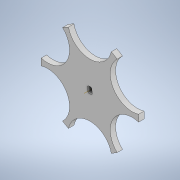
# Autodesk Inventor part: шестеренка_для_мозговорота
Saved by Autodesk Inventor 2021.1 (Build 251245010, 245A)
## iProperties
Created: 2022-11-11
Part Number: шестеренка_для_мозговорота
Material: Типовые
Document SubType Name: Modeling
Designer: zmoze
Density: 1 g/cm^3
Appearance: По умолчанию
Author: zmoze
Autodesk Inventor part; units mm, degrees
ref_plane "YZ Plane" through (0, 0, 0) normal (1, 0, 0) x (0, 1, 0)
ref_plane "XZ Plane" through (0, 0, 0) normal (0, 1, 0) x (-1, 0, 0)
sketch "Эскиз1" plane through (0, 0, 0) normal (0, 0, 1) x (1, 0, 0)
  arc A0 (-19.7308, 40.4437) -> (19.7308, 40.4437) centre (0, 0) ccw
  circle A1 centre (0, 45) radius 20.25
  line L0 (0, 91.35) -> (0, -91.35) projected
  circle A2 centre (-38.9711, 22.5) radius 20.25
  circle A3 centre (-38.9711, -22.5) radius 20.25
  circle A4 centre (0, -45) radius 20.25
  circle A5 centre (38.9711, -22.5) radius 20.25
  circle A6 centre (38.9711, 22.5) radius 20.25
  point P0 (-19.7308, -40.4437)
  point P1 (19.7308, -40.4438)
  point P2 (25.1599, -37.3092)
  point P3 (44.8907, -3.1345)
  point P4 (44.8907, 3.1345)
  point P5 (25.1599, 37.3092)
  point P6 (-25.1599, 37.3092)
  point P7 (-44.8907, 3.1345)
  point P8 (-44.8907, -3.1345)
  point P9 (-25.1599, -37.3092)
  dimension "d0" = 40.5
  dimension "d3" = 360
  dimension "d5" = 90
  constraints: 7 centre point, 5 point on circle, 2 coincident, 1 point on line, 13 other
  measures "d0" diameter of A1
  measures "d5" diameter of A0
extrude "Выдавливание1" add sketch "Эскиз1" along normal blind 5 contours A1 L0 A4 A0 A3 A2 | A1 A0 A6 A5 A4 L0
sketch "Эскиз2" plane through (0, 0, 5) normal (0, 0, 1) x (1, 0, 0)
  line L0 (-1.3319, -1.492) -> (-1.6468, 1.135) projected
  arc A0 (-1.2513, -2.1643) -> (1.7273, -1.8073) centre (0, 0) ccw projected
  line L1 (1.3319, 1.492) -> (1.6468, -1.135) projected
  line L2 (-1.2513, -2.1643) -> (-1.3319, -1.492) projected
  line L3 (1.6468, -1.135) -> (1.7273, -1.8073) projected
  arc A1 (1.2513, 2.1643) -> (-1.7273, 1.8073) centre (0, 0) ccw projected
  line L4 (1.2513, 2.1643) -> (1.3319, 1.492) projected
  line L5 (-1.6468, 1.135) -> (-1.7273, 1.8073) projected
  arc A2 (1.7197, 2.4582) -> (-2.2519, 1.9822) centre (0, 0) ccw
  line L6 (1.7197, 2.4582) -> (2, 0.1194)
  line L7 (2, 0.1194) -> (1.9988, 0.1295)
  line L8 (1.9988, 0.1295) -> (2.2519, -1.9822)
  arc A3 (-1.7197, -2.4582) -> (2.2519, -1.9822) centre (0, 0) ccw
  line L9 (-1.7197, -2.4582) -> (-1.9735, -0.3403)
  line L10 (-1.9735, -0.3403) -> (-1.9716, -0.3566)
  line L11 (-1.9716, -0.3566) -> (-2.2519, 1.9822)
  point P0 (0, 0)
  point P1 (-1.9716, -0.3566)
  point P2 (2, 0.1296)
  dimension "d8" = 0.5
  constraints: 12 end point, 4 point on circle, 2 centre point, 7 other
  measures "d8" distance between parallel lines of L7 L1
extrude "Выдавливание2" cut sketch "Эскиз2" against normal through all contours L0 L5 A1 L4 L1 L3 A0 L2 | L6 L8 A3 L9 L11 A2
ref_plane "РабПлоскость1" through (0, 0, 2.5) normal (0, 0, 1) x (1, 0, 0)
